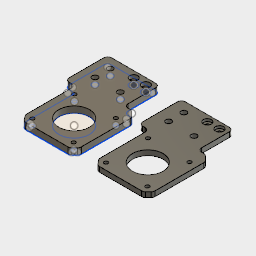
Y_Motor_Bracket_v2 (Autodesk Fusion 360 design; units mm, degrees)
Autodesk Fusion 360 part; units mm, degrees
sketch "Sketch1" plane through (0, 0, 0) normal (0, 1, 0) x (1, 0, 0)
  line L0 (-22, 1) -> (-22, -36.9477)
  line L1 (-21.3426, -38.8217) -> (-18.9007, -41.8741)
  line L2 (-16.5581, -43) -> (16.7574, -43)
  line L3 (18.8787, -42.1213) -> (21.1213, -39.8787)
  line L4 (22, -37.7574) -> (22, 0.7574)
  line L5 (21.1213, 2.8787) -> (17.8787, 6.1213)
  line L6 (15.7574, 7) -> (14, 7)
  line L7 (11, 10) -> (11, 32)
  line L8 (8, 35) -> (-27, 35)
  line L9 (-30, 32) -> (-30, 4.5)
  line L10 (-27, 1.5) -> (-25, 1.5)
  line L11 (-22, -1.5) -> (-22, 1)
  arc A0 (-27, 35) -> (-30, 32) centre (-27, 32) ccw
  arc A1 (11, 32) -> (8, 35) centre (8, 32) ccw
  arc A2 (11, 10) -> (14, 7) centre (14, 10) ccw
  arc A3 (17.8787, 6.1213) -> (15.7574, 7) centre (15.7574, 4) ccw
  arc A4 (22, 0.7574) -> (21.1213, 2.8787) centre (19, 0.7574) ccw
  arc A5 (21.1213, -39.8787) -> (22, -37.7574) centre (19, -37.7574) ccw
  arc A6 (16.7574, -43) -> (18.8787, -42.1213) centre (16.7574, -40) ccw
  arc A7 (-18.9007, -41.8741) -> (-16.5581, -43) centre (-16.5581, -40) ccw
  arc A8 (-22, -36.9477) -> (-21.3426, -38.8217) centre (-19, -36.9477) ccw
  arc A9 (-22, -1.5) -> (-25, 1.5) centre (-25, -1.5) ccw
  arc A10 (-30, 4.5) -> (-27, 1.5) centre (-27, 4.5) ccw
  circle A11 centre (-0.2984, -21.1128) radius 12.0091
  circle A12 centre (-16.6117, -4.559) radius 1.5
  circle A13 centre (15.9625, -4.5108) radius 1.5
  circle A14 centre (15.9625, -37.6823) radius 1.5
  circle A15 centre (-16.5593, -37.7148) radius 1.5
  circle A16 centre (-20, 15) radius 2.2361
  circle A17 centre (0, 15) radius 2.2361
  circle A18 centre (-20, 27) radius 2.2
  circle A19 centre (-4.4645, 29.9673) radius 3.1135
  circle A20 centre (5.1514, 29.9363) radius 3.1428
  circle A21 centre (-4.4645, 29.9673) radius 1.0248
  circle A22 centre (5.1514, 29.9363) radius 1.0442
  dimension "d1" = 3
  dimension "d2" = 3
  dimension "d3" = 3
  dimension "d4" = 3
  dimension "d5" = 3
  dimension "d6" = 4.4
  measures "d1" radius of A0
  measures "d2" diameter of A12
  measures "d3" diameter of A13
  measures "d4" diameter of A14
  measures "d5" diameter of A15
  measures "d6" diameter of A18
extrude "Extrude1" add sketch "Sketch1" along normal blind 5 contours L0 L1 L2 L3 L4 L5 L6 L7 L8 L9 L10 A0 A1 A2 A3 A4 A5 A6 A7 A8 A9 A10 makes body 1
extrude "Extrude2" add sketch "Sketch1" along normal blind 2 contours A19 | A20 bodies 1
copy_body "CopyPasteBodies1" bodies 1 makes body 2
move_body "Move1" bodies 2 to x (1, 0, 0) y (0, 1, 0) z (0, 0, 1) at (58, 0, 0)
move_face "OffsetFaces1" offset -1 1 faces at (46.0461, 5, -7.8994) on bodies 2
named bodies: "5mm", "4mm"
